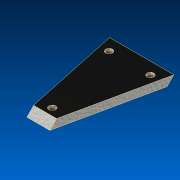
# Autodesk Inventor part: triangular
Saved by Autodesk Inventor 2016 (Build 200138000, 138)
## iProperties
Created: 2018-12-07
Part Number: triangular
Material: Generic
Document SubType Name: Modeling
Designer: lesly
Density: 1 g/cm^3
Appearance: Nickel
Author: lesly
Autodesk Inventor part; units mm, degrees
sketch "Sketch1" plane through (0, 0, 0) normal (1, 0, 0) x (0, 1, 0)
  line L0 (-28.3154, 9.9073) -> (-28.3154, -18.0927)
  line L1 (13.6846, -4.0927) -> (13.6846, -9.0927)
  line L2 (13.6846, -4.0927) -> (13.6846, 0.9073)
  line L3 (-28.3154, 9.9073) -> (13.6846, 0.9073)
  line L4 (-28.3154, -18.0927) -> (13.6846, -9.0927)
  point P0 (0, 0)
  constraints: 10 end point
ref_plane "Work Plane2" through (1, 0, 0) normal (1, 0, 0) x (0, 1, 0)
sketch "Sketch5" plane through (1, 0, 0) normal (1, 0, 0) x (0, 1, 0)
  line L0 (-29.3154, 9.9073) -> (12.6846, 0.9073)
  line L1 (12.6846, -4.0927) -> (12.6846, 0.9073)
  line L2 (12.6846, -4.0927) -> (12.6846, -9.0927)
  line L3 (-29.3154, -18.0927) -> (12.6846, -9.0927)
  line L4 (-29.3154, 9.9073) -> (-29.3154, -18.0927)
  point P0 (0, 0)
  constraints: 10 end point
loft "Loft1" add profiles "Sketch1", "Sketch5"
ref_plane "Work Plane8" through (2, 0, 0) normal (1, 0, 0) x (0, 1, 0)
sketch "Sketch8" plane through (2, 0, 0) normal (1, 0, 0) x (0, 1, 0)
  line L0 (-30.3154, 9.9073) -> (11.6846, 0.9073)
  line L1 (11.6846, -9.0927) -> (-30.3154, -18.0927)
  line L2 (-30.3154, -18.0927) -> (-30.3154, 9.9073)
  line L3 (11.6846, 0.9073) -> (11.6846, -9.0927)
  point P0 (0, 0)
  constraints: 8 end point, 1 vertical
loft "Loft2" add profiles "Sketch8" section 1 edges at (1, -29.3154, -4.0927) (1, -8.3154, -13.5927) (1, 12.6846, -6.5927) (1, 12.6846, -1.5927) (1, -8.3154, 5.4073)
ref_plane "Work Plane6" through (3, 0, 0) normal (1, 0, 0) x (0, 1, 0)
sketch "Sketch9" plane through (3, 0, 0) normal (1, 0, 0) x (0, 1, 0)
  line L0 (-31.3154, 9.9073) -> (-31.3154, -18.0927)
  line L1 (-31.3154, -18.0927) -> (10.6846, -9.0927)
  line L2 (10.6846, -9.0927) -> (10.6846, 0.9073)
  line L3 (10.6846, 0.9073) -> (-31.3154, 9.9073)
  line L4 (11.6846, -9.0927) -> (11.6846, 0.9073) projected
  point P0 (-1, 0)
  constraints: 8 end point
loft "Loft3" add profiles "Sketch9" section 1 edges at (2, -30.3154, -4.0927) (2, -9.3154, -13.5927) (2, 11.6846, -4.0927) (2, -9.3154, 5.4073)
sketch "Sketch10" plane through (3, -31.3154, 9.9073) normal (1, 0, 0) x (0, 0, -1)
  circle A0 centre (5, 5.2079) radius 1
  circle A1 centre (23, 5.2079) radius 1
  circle A2 centre (14, 38.9079) radius 1
  point P0 (9.9073, 31.3154)
  dimension "d36" = 33.7
  dimension "d37" = 33.7
  dimension "d38" = 18
  dimension "d39" = 9
  constraints: 3 centre point, 3 coincident, 1 other
  measures "d36" vertical distance of A0.centre A2.centre
  measures "d37" vertical distance of A2.centre A1.centre
  measures "d38" distance of A0.centre A1.centre
  measures "d39" horizontal distance of A2.centre A1.centre
extrude "Extrusion1" cut sketch "Sketch10" against normal blind 3
chamfer "Chamfer1" distance 0.5 angle 45 1 edges at (3, -26.1075, 5.9073)
chamfer "Chamfer2" distance 0.5 angle 45 2 edges at (3, -26.1075, -12.0927) (3, 7.5925, -3.0927)
body "Solid1"
